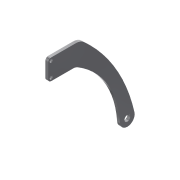
# Autodesk Inventor part: handle_top
Saved by Autodesk Inventor 2018 (Build 220112000, 112)
## iProperties
Created: 2018-09-01
Part Number: handle_top
Material: 一般
Document SubType Name: Modeling
Designer: y6tada
Density: 1 g/cm^3
Appearance: 機械加工 - アルミニウム
Author: y6tada
Autodesk Inventor part; units mm, degrees
ref_plane "YZ Plane" through (0, 0, 0) normal (1, 0, 0) x (0, 1, 0)
ref_plane "XZ Plane" through (0, 0, 0) normal (0, 1, 0) x (-1, 0, 0)
ref_plane "XY Plane" through (0, 0, 0) normal (0, 0, 1) x (1, 0, 0)
sketch "スケッチ1" plane through (0, 0, 0) normal (1, 0, 0) x (0, 1, 0)
  line L0 (0, 5) -> (0, -5) construction
  circle A0 centre (0, 5) radius 1.05
  circle A1 centre (0, -5) radius 1.05
  line L1 (17, 7) -> (0, 7)
  line L2 (-2, 5) -> (-2, -5)
  line L3 (0, -7) -> (15, -7)
  arc A2 (47.0107, -55.3275) -> (56.875, -53.8889) centre (52, -55) ccw
  arc A3 (56.875, -53.8889) -> (22.3567, 4.9418) centre (-53.3232, -79.0044) ccw
  arc A4 (22.3567, 4.9418) -> (17, 7) centre (17, -1) ccw
  arc A5 (47.0107, -55.3275) -> (18.0956, -7.8602) centre (-12.8604, -59.258) ccw
  arc A6 (18.0956, -7.8602) -> (15, -7) centre (15, -13) ccw
  arc A7 (0, 7) -> (-2, 5) centre (0, 5) ccw
  arc A8 (-2, -5) -> (0, -7) centre (0, -5) ccw
  circle A9 centre (52, -55) radius 2
  arc A10 (55.0761, -62.1956) -> (42.6675, -20.0067) centre (-12.8604, -59.258) ccw construction
  point P0 (0, 0)
  point P1 (0, 0)
  dimension "d0" = 2.1
  dimension "d2" = 2
  dimension "d3" = 4
  dimension "d4" = 5
  dimension "d5" = 15
  dimension "d6" = 6
  dimension "d8" = 8
  dimension "d10" = 55
  dimension "d11" = 8
  dimension "d12" = 60
  dimension "d24" = 2
  dimension "d25" = 14
  dimension "d26" = 35
  constraints: 16 point on circle, 11 centre point, 11 tangent, 8 end point, 4 coincident, 3 concentric, 2 equal radius, 2 perpendicular, 1 horizontal, 1 midpoint, 1 vertical
  measures "d0" diameter of A1
  measures "d2" radius of A7
  measures "d3" diameter of A9
  measures "d4" radius of A2
  measures "d5" distance from line of A6.centre L0
  measures "d6" radius of A6
  measures "d8" radius of A4
  measures "d10" vertical distance of point (0, 0) A2.centre
  measures "d11" radial gap between concentric circles of A5 A10
  measures "d12" radius of A5
  measures "d24" horizontal distance of A4.centre A6.centre
  measures "d25" distance between parallel lines of L3 L1
  measures "d26" horizontal distance of A2.centre A4.centre
extrude "押し出し1" add sketch "スケッチ1" along normal blind 2
